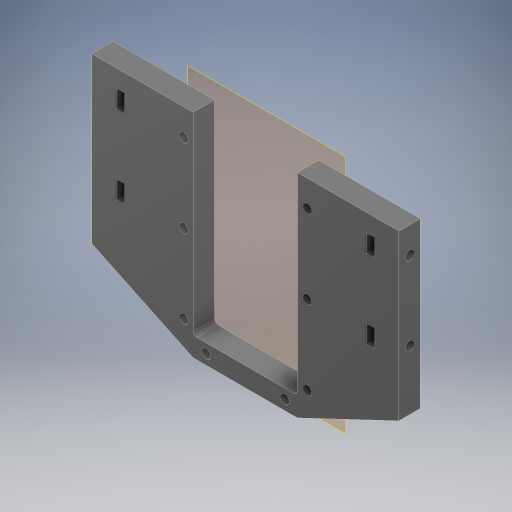
# Autodesk Inventor part: connecting plate under body
Saved by Autodesk Inventor 2024 (Build 280153000, 153)
## iProperties
Created: 2024-09-03
Part Number: connecting plate under body
Material: PMMA 플라스틱
Document SubType Name: Modeling
Designer: msi
Density: 1.188 g/cm^3
Appearance: 매끄러움 - 검은색
Mass: 8.88706 g
Surface Area: 39.037 cm^2
Volume: 7.48069 cm^3
Author: msi
Autodesk Inventor part; units mm, degrees
ref_plane "YZ Plane" through (0, 0, 0) normal (1, 0, 0) x (0, 1, 0)
ref_plane "XZ Plane" through (0, 0, 0) normal (0, 1, 0) x (-1, 0, 0)
ref_plane "XY Plane" through (0, 0, 0) normal (0, 0, 1) x (1, 0, 0)
ref_plane "작업 평면1" through (0, 0, 0) normal (0, 0, 1) x (1, 0, 0)
sketch "스케치1" plane through (0, 0, 0) normal (0, 0, 1) x (1, 0, 0)
  arc A0 (20.1, 4.5766) -> (19.5808, 6.2636) centre (17.1, 4.5766) ccw projected
  line L0 (19.5808, 6.2636) -> (15.5953, 12.1246) projected
  arc A1 (15.5953, 12.1246) -> (13.9414, 13) centre (13.9414, 11) ccw projected
  line L1 (13, 13) -> (13.9414, 13) projected
  arc A2 (14.5, 11.5) -> (13, 13) centre (13, 11.5) ccw projected
  line L2 (14.5, -41.5) -> (14.5, 11.5) projected
  arc A3 (13.5, -42.5) -> (14.5, -41.5) centre (13.5, -41.5) ccw projected
  line L3 (-13.5, -42.5) -> (13.5, -42.5) projected
  arc A4 (-14.5, -41.5) -> (-13.5, -42.5) centre (-13.5, -41.5) ccw projected
  line L4 (-14.5, 11.5) -> (-14.5, -41.5) projected
  arc A5 (-13, 13) -> (-14.5, 11.5) centre (-13, 11.5) ccw projected
  line L5 (-13.9414, 13) -> (-13, 13) projected
  arc A6 (-13.9414, 13) -> (-15.5953, 12.1246) centre (-13.9414, 11) ccw projected
  line L6 (-15.5953, 12.1246) -> (-19.5808, 6.2636) projected
  arc A7 (-19.5808, 6.2636) -> (-20.1, 4.5766) centre (-17.1, 4.5766) ccw projected
  line L7 (-20.1, 4.5766) -> (-20.1, -39.6766) projected
  arc A8 (-20.1, -39.6766) -> (-19.5808, -41.3636) centre (-17.1, -39.6766) ccw projected
  line L8 (-19.5808, -41.3636) -> (-15.8929, -46.7869) projected
  arc A9 (-15.8929, -46.7869) -> (-13.4121, -48.1) centre (-13.4121, -45.1) ccw projected
  line L9 (-13.4121, -48.1) -> (13.4121, -48.1) projected
  arc A10 (13.4121, -48.1) -> (15.8929, -46.7869) centre (13.4121, -45.1) ccw projected
  line L10 (15.8929, -46.7869) -> (19.5808, -41.3636) projected
  arc A11 (19.5808, -41.3636) -> (20.1, -39.6766) centre (17.1, -39.6766) ccw projected
  line L11 (20.1, -39.6766) -> (20.1, 4.5766) projected
  circle A12 centre (-17.3, 4) radius 1.35 projected
  circle A13 centre (-17.3, -18) radius 1.35 projected
  circle A14 centre (-11, -45.3) radius 1.35 projected
  circle A15 centre (17.3, 4) radius 1.35 projected
  circle A16 centre (17.3, -18) radius 1.35 projected
  circle A17 centre (11, -45.3) radius 1.35 projected
  circle A18 centre (-17.3, -40) radius 1.35 projected
  circle A19 centre (17.3, -40) radius 1.35 projected
  arc A20 (14.6, 11.5) -> (12.2254, 12.9) centre (13, 11.5) ccw
  line L12 (12.2254, 12.9) -> (13.9414, 12.9)
  arc A21 (15.5126, 12.0684) -> (13.9414, 12.9) centre (13.9414, 11) ccw
  line L13 (15.5126, 12.0684) -> (15.8991, 11.5)
  line L14 (19.3671, -41.5) -> (15.8102, -46.7307)
  arc A22 (13.4121, -48) -> (15.8102, -46.7307) centre (13.4121, -45.1) ccw
  line L15 (13.4121, -48) -> (-13.4121, -48)
  arc A23 (-15.8102, -46.7307) -> (-13.4121, -48) centre (-13.4121, -45.1) ccw
  line L16 (-15.8102, -46.7307) -> (-19.4981, -41.3073)
  arc A24 (-20, -39.6766) -> (-19.4981, -41.3073) centre (-17.1, -39.6766) ccw
  line L17 (-20, -39.6766) -> (-20, 4.5766)
  arc A25 (-19.4981, 6.2073) -> (-20, 4.5766) centre (-17.1, 4.5766) ccw
  line L18 (-19.4981, 6.2073) -> (-15.5126, 12.0684)
  arc A26 (-13.9414, 12.9) -> (-15.5126, 12.0684) centre (-13.9414, 11) ccw
  line L19 (-13.9414, 12.9) -> (-12.2254, 12.9)
  arc A27 (-12.2254, 12.9) -> (-14.6, 11.5) centre (-13, 11.5) ccw
  line L20 (-14.6, 11.5) -> (-14.6, -41.5)
  arc A28 (-14.6, -41.5) -> (-13.5, -42.6) centre (-13.5, -41.5) ccw
  line L21 (-13.5, -42.6) -> (13.5, -42.6)
  arc A29 (13.5, -42.6) -> (14.6, -41.5) centre (13.5, -41.5) ccw
  line L22 (14.6, -41.5) -> (14.6, 11.5)
  line L23 (14.6, 11.5) -> (39.6, 11.5)
  line L24 (39.6, -41.5) -> (14.6, -41.5)
  line L25 (14.6, -41.5) -> (14.6, 11.5)
  circle A30 centre (17.3, 4) radius 1.35
  circle A31 centre (17.3, -18) radius 1.35
  line L26 (45.5, -39.6766) -> (45.5, -37.525) projected
  line L27 (47.5, -37.525) -> (45.5, -37.525) projected
  line L28 (47.5, -36.025) -> (47.5, -37.525) projected
  line L29 (47.5, -36.025) -> (45, -36.025) projected
  line L30 (45, -36.025) -> (45, -21.975) projected
  line L31 (47.5, -21.975) -> (45, -21.975) projected
  line L32 (47.5, -21.975) -> (47.5, -20.475) projected
  line L33 (47.5, -20.475) -> (45.5, -20.475) projected
  line L34 (45.5, -20.475) -> (45.5, -15.525) projected
  line L35 (47.5, -15.525) -> (45.5, -15.525) projected
  line L36 (47.5, -15.525) -> (47.5, -14.025) projected
  line L37 (47.5, -14.025) -> (45, -14.025) projected
  line L38 (45, -14.025) -> (45, 0.025) projected
  line L39 (47.5, 0.025) -> (45, 0.025) projected
  line L40 (47.5, 0.025) -> (47.5, 1.525) projected
  line L41 (47.5, 1.525) -> (45.5, 1.525) projected
  line L42 (45.5, 1.525) -> (45.5, 4.5766) projected
  line L43 (43, 4.5766) -> (45.5, 4.5766) projected
  line L44 (43, -39.6766) -> (43, 4.5766) projected
  line L45 (43, -39.6766) -> (45.5, -39.6766) projected
  line L46 (14.6, 11.5) -> (43, 11.5)
  line L47 (43, 11.5) -> (43, -41.5)
  line L48 (43, -41.5) -> (14.6, -41.5)
  line L49 (14.6, -41.5) -> (14.6, 11.5)
  line L50 (45.5, -19.35) -> (45.5, -16.65) projected
  line L51 (43, -19.35) -> (43, -16.65) projected
  line L52 (43, -19.35) -> (43, -16.65) projected
  line L53 (43, -19.35) -> (43, -16.65) projected
  line L54 (47.5, -18) -> (45.5, -18) projected
  line L55 (47.5, 4) -> (45.5, 4) projected
  line L56 (33.5, 1) -> (36.5, 7) construction
  line L57 (36.5, 1) -> (33.5, 7) construction
  line L58 (33.9, 1.4) -> (36.1, 6.6) construction
  point P0 (0, 0)
  point P1 (19.488, -41.5)
  point P2 (16.02, 11.5)
  dimension "d0" = 0.1
  dimension "d1" = 25
  dimension "d2" = 53
  dimension "d3" = 2.7
  dimension "d4" = 2.7
  dimension "d5" = 3
  dimension "d6" = 6
  constraints: 42 end point, 20 point on circle, 12 centre point, 3 parallel, 2 coincident, 2 horizontal, 2 point on line, 1 perpendicular, 17 other
  measures "d0" distance between parallel lines of L2 L22
  measures "d1" distance of L24.start L24.end
  measures "d2" distance of L23.end L24.start
  measures "d3" diameter of A30
  measures "d4" diameter of A31
  measures "d5" distance of L57.end L56.end
  measures "d6" distance of L56.end L57.start
extrude "돌출4" add sketch "스케치1" along normal blind 6 contours L11 A11 L10 L24 L22 L23 L0 A0 | A0 L0 L23 L46 L47 L44 L48 L24 L10 A11 L11 | A19
sketch "스케치3" plane through (43, -41.5, 0) normal (1, 0, 0) x (0, 0, -1)
  arc A0 (-5.0808, 47.7636) -> (-5.6, 46.0766) centre (-2.6, 46.0766) ccw projected
  line L0 (-5.6, 1.8234) -> (-5.6, 46.0766) projected
  arc A1 (-5.6, 1.8234) -> (-5.0808, 0.1364) centre (-2.6, 1.8234) ccw projected
  line L1 (-1.3929, -5.2869) -> (-5.0808, 0.1364) projected
  arc A2 (-1.3929, -5.2869) -> (1.0879, -6.6) centre (1.0879, -3.6) ccw projected
  line L2 (27.9121, -6.6) -> (1.0879, -6.6) projected
  arc A3 (27.9121, -6.6) -> (30.3929, -5.2869) centre (27.9121, -3.6) ccw projected
  line L3 (34.0808, 0.1364) -> (30.3929, -5.2869) projected
  arc A4 (34.0808, 0.1364) -> (34.6, 1.8234) centre (31.6, 1.8234) ccw projected
  line L4 (34.6, 46.0766) -> (34.6, 1.8234) projected
  arc A5 (34.6, 46.0766) -> (34.0808, 47.7636) centre (31.6, 46.0766) ccw projected
  line L5 (30.0953, 53.6246) -> (34.0808, 47.7636) projected
  arc A6 (30.0953, 53.6246) -> (28.4414, 54.5) centre (28.4414, 52.5) ccw projected
  line L6 (22.15, 54.5) -> (28.4414, 54.5) projected
  arc A7 (23.65, 53) -> (22.15, 54.5) centre (22.15, 53) ccw projected
  line L7 (23.65, 53) -> (23.65, 51.5) projected
  arc A8 (23.65, 51.5) -> (26, 49.15) centre (26, 51.5) ccw projected
  line L8 (26, 49.15) -> (28, 49.15) projected
  arc A9 (29, 48.15) -> (28, 49.15) centre (28, 48.15) ccw projected
  line L9 (29, 48.15) -> (29, 5.35) projected
  arc A10 (28, 4.35) -> (29, 5.35) centre (28, 5.35) ccw projected
  line L10 (28, 4.35) -> (26, 4.35) projected
  arc A11 (26, 4.35) -> (23.65, 2) centre (26, 2) ccw projected
  line L11 (23.65, 2) -> (23.65, 0) projected
  arc A12 (22.65, -1) -> (23.65, 0) centre (22.65, 0) ccw projected
  line L12 (22.65, -1) -> (6.35, -1) projected
  arc A13 (5.35, 0) -> (6.35, -1) centre (6.35, 0) ccw projected
  line L13 (5.35, 0) -> (5.35, 2) projected
  arc A14 (5.35, 2) -> (3, 4.35) centre (3, 2) ccw projected
  line L14 (3, 4.35) -> (1, 4.35) projected
  arc A15 (0, 5.35) -> (1, 4.35) centre (1, 5.35) ccw projected
  line L15 (0, 5.35) -> (0, 48.15) projected
  arc A16 (1, 49.15) -> (0, 48.15) centre (1, 48.15) ccw projected
  line L16 (1, 49.15) -> (3, 49.15) projected
  arc A17 (3, 49.15) -> (5.35, 51.5) centre (3, 51.5) ccw projected
  line L17 (5.35, 51.5) -> (5.35, 53) projected
  arc A18 (6.85, 54.5) -> (5.35, 53) centre (6.85, 53) ccw projected
  line L18 (0.5586, 54.5) -> (6.85, 54.5) projected
  arc A19 (0.5586, 54.5) -> (-1.0953, 53.6246) centre (0.5586, 52.5) ccw projected
  line L19 (-5.0808, 47.7636) -> (-1.0953, 53.6246) projected
  circle A20 centre (31.8, 45.5) radius 1.35 projected
  circle A21 centre (31.8, 23.5) radius 1.35 projected
  circle A22 centre (25.5, -3.8) radius 1.35 projected
  circle A23 centre (-2.8, 45.5) radius 1.35 projected
  circle A24 centre (-2.8, 23.5) radius 1.35 projected
  circle A25 centre (3.5, -3.8) radius 1.35 projected
  circle A26 centre (31.8, 1.5) radius 1.35 projected
  circle A27 centre (-2.8, 1.5) radius 1.35 projected
  circle A28 centre (-2.8, 45.5) radius 1.35
  circle A29 centre (-2.8, 23.5) radius 1.35
  point P0 (0, 41.5)
  constraints: 2 centre point, 2 coincident, 2 concentric
extrude "돌출5" cut sketch "스케치3" against normal blind 15 contours A23 | A24
sketch "스케치4" plane through (0, 0, 6) normal (0, 0, 1) x (1, 0, 0)
  line L0 (36.1, 1.4) -> (33.9, 1.4)
  line L1 (33.9, 1.4) -> (33.9, 6.6)
  line L2 (33.9, 6.6) -> (36.1, 6.6)
  line L3 (36.1, 6.6) -> (36.1, 1.4)
  line L4 (36.1, 1.4) -> (33.9, 6.6) construction
  line L5 (33.9, 1.4) -> (36.1, 6.6) construction
  line L6 (43, -16.65) -> (28, -16.65) projected
  line L7 (43, -19.35) -> (28, -19.35) projected
  line L8 (33.9, -20.6) -> (36.1, -20.6)
  line L9 (36.1, -20.6) -> (36.1, -15.4)
  line L10 (36.1, -15.4) -> (33.9, -15.4)
  line L11 (33.9, -15.4) -> (33.9, -20.6)
  line L12 (33.9, -20.6) -> (36.1, -15.4) construction
  line L13 (36.1, -20.6) -> (33.9, -15.4) construction
  point P0 (0, 0)
  point P1 (35, 4)
  point P2 (35, -18)
  dimension "d22" = 2.2
  dimension "d23" = 5.2
  dimension "d24" = 2.2
  dimension "d25" = 5.2
  constraints: 24 end point, 4 midpoint, 4 parallel, 2 horizontal, 2 perpendicular
  measures "d22" distance of L1.end L2.end
  measures "d23" distance of L0.end L1.end
  measures "d24" distance of L10.end L9.end
  measures "d25" distance of L9.end L8.end
extrude "돌출6" cut sketch "스케치4" against normal blind 6
sketch "스케치5" plane through (0, 0, 6) normal (0, 0, 1) x (1, 0, 0)
  line L0 (33.9, 1.4) -> (33.9, 6.6) projected
  line L1 (33.9, 6.6) -> (36.1, 6.6) projected
  line L2 (36.1, 6.6) -> (36.1, 1.4) projected
  line L3 (36.1, 1.4) -> (33.9, 1.4) projected
  line L4 (36.1, -20.6) -> (33.9, -20.6) projected
  line L5 (33.9, -20.6) -> (33.9, -15.4) projected
  line L6 (33.9, -15.4) -> (36.1, -15.4) projected
  line L7 (36.1, -15.4) -> (36.1, -20.6) projected
  line L8 (14.6, -41.5) -> (43, -41.5) projected
  line L9 (43, -41.5) -> (43, 11.5) projected
  line L10 (43, 11.5) -> (14.6, 11.5) projected
  line L11 (14.6, 11.5) -> (14.6, -41.5) projected
  circle A0 centre (17.3, 4) radius 1.35 projected
  circle A1 centre (17.3, -18) radius 1.35 projected
  line L12 (43, -41.5) -> (14.6, -41.5)
  line L13 (14.6, -41.5) -> (14.6, -34.5)
  line L14 (14.6, -34.5) -> (43, -34.5)
  line L15 (43, -34.5) -> (43, -41.5)
  point P0 (0, 0)
  dimension "d28" = 7
  constraints: 8 end point, 2 parallel, 1 horizontal, 1 perpendicular, 1 point on line
  measures "d28" distance of L12.end L13.end
extrude "돌출7" cut sketch "스케치5" against normal blind 10 contours L11 L14 L9 L8
sketch "스케치7" plane through (0, 0, 6) normal (0, 0, 1) x (1, 0, 0)
  circle A0 centre (17.3, -40) radius 1.35
  circle A1 centre (11, -45.3) radius 1.35
  circle A2 centre (-11, -45.3) radius 1.35
  circle A3 centre (-17.3, -40) radius 1.35
  line L0 (-13.4121, -48.1) -> (13.4121, -48.1)
  line L1 (-13, -42.5) -> (13, -42.5)
  line L2 (20.1, -39.6766) -> (20.1, 4.5766)
  line L3 (14.5, -41) -> (14.5, 11)
  line L4 (14.6, 11.5) -> (14.6, -34.5) projected
  line L5 (14.6, -34.5) -> (43, -34.5) projected
  line L6 (20, -39.6766) -> (20, 4.5766)
  line L7 (14.6, -41) -> (14.6, 11)
  line L8 (-13, -42.6) -> (13, -42.6)
  line L9 (-13.4121, -48) -> (13.4121, -48)
  line L10 (14.6, -34.5) -> (20, -34.5)
  line L11 (20, -34.5) -> (20, -42.6)
  line L12 (14.6, -42.6) -> (14.6, -34.5)
  line L13 (14.6, -42.6) -> (0, -42.6)
  line L14 (0, -42.6) -> (0, -48)
  line L15 (0, -48) -> (14.6, -48)
  line L16 (20, -42.6) -> (14.6, -48)
  circle A4 centre (17.3, -40) radius 1.35
  circle A5 centre (11, -45.3) radius 1.35
  point P0 (0, 0)
  point P1 (41, -34.5)
  point P2 (20, -34.5)
  point P3 (13, -42.6)
  point P4 (0, -42.6)
  point P5 (13.4121, -48)
  dimension "d33" = 0.1
  dimension "d35" = 0.1
  dimension "d36" = 0.1
  dimension "d37" = 0.1
  constraints: 30 end point, 6 centre point, 6 parallel, 4 horizontal, 2 coincident, 2 concentric, 2 perpendicular, 2 vertical, 1 midpoint, 16 other
  measures "d33" distance between parallel lines of L2 L6
  measures "d35" distance between parallel lines of L3 L7
  measures "d36" distance between parallel lines of L1 L8
  measures "d37" distance between parallel lines of L0 L9
extrude "돌출8" add sketch "스케치7" against normal blind 6 contours L5 L6 L11 L16 L15 L9 L14 L8 L13 L12 L7
fillet "모깎기5" radius 1 1 edges at (14.6, -42.6, 3)
sketch "스케치8" plane through (0, 0, 6) normal (0, 0, 1) x (1, 0, 0)
  circle A0 centre (11, -45.3) radius 1.35 projected
  circle A1 centre (17.3, -40) radius 1.35 projected
  circle A2 centre (17.3, -18) radius 1.35 projected
  circle A3 centre (17.3, 4) radius 1.35 projected
  line L0 (36.1, -20.6) -> (33.9, -20.6) projected
  line L1 (33.9, -20.6) -> (33.9, -15.4) projected
  line L2 (33.9, -15.4) -> (36.1, -15.4) projected
  line L3 (36.1, -15.4) -> (36.1, -20.6) projected
  line L4 (33.9, 1.4) -> (33.9, 6.6) projected
  line L5 (33.9, 6.6) -> (36.1, 6.6) projected
  line L6 (36.1, 6.6) -> (36.1, 1.4) projected
  line L7 (36.1, 1.4) -> (33.9, 1.4) projected
  line L8 (14.6, -48) -> (20, -42.6) projected
  line L9 (20, -42.6) -> (20, -34.5) projected
  line L10 (20, -34.5) -> (43, -34.5) projected
  line L11 (43, -34.5) -> (43, 11.5) projected
  line L12 (43, 11.5) -> (14.6, 11.5) projected
  line L13 (14.6, 11.5) -> (14.6, -41.6) projected
  arc A4 (13.6, -42.6) -> (14.6, -41.6) centre (13.6, -41.6) ccw projected
  line L14 (13.6, -42.6) -> (0, -42.6) projected
  line L15 (0, -48) -> (14.6, -48) projected
  line L16 (0, -42.6) -> (0, -48) projected
  line L17 (43, -34.5) -> (19.4142, -34.5)
  line L18 (19.4142, -34.5) -> (19.4142, -43.1858)
  line L19 (14.6, -48) -> (43, -34.5)
  line L20 (19.4142, -43.1858) -> (14.6, -48)
  point P0 (0, 0)
  constraints: 8 end point, 2 point on line, 1 collinear
extrude "돌출12" add sketch "스케치8" against normal blind 6 contours L8 L9 L10 L19
mirror "미러2" about plane through (0, -48, 6) normal (-1, 0, 0)
